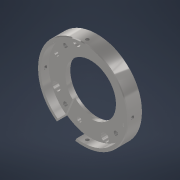
# Autodesk Inventor part: 006
Saved by Autodesk Inventor 2022 (Build 260153000, 153)
## iProperties
Created: 2021-11-05
Part Number: 006
Material: Stainless Steel, 440C
Document SubType Name: Modeling
Designer: vinicius.miguel
Density: 7.75 g/cm^3
Appearance: Semi-Polished
Mass: 959.118 g
Surface Area: 466.738 cm^2
Volume: 123.757 cm^3
Author: vinicius.miguel
Autodesk Inventor part; units mm, degrees
ref_plane "XY Plane" through (0, 0, 0) normal (0, 0, 1) x (1, 0, 0)
sketch "Sketch1" plane through (0, 0, 0) normal (0, 1, 0) x (-1, 0, 0)
  line L0 (0, 0) -> (0, -51.1103) construction
  line L1 (-37.5, -17) -> (-40, -17)
  line L2 (-40, -17) -> (-40, -22)
  line L3 (-40, -22) -> (-67, -22)
  line L4 (-67, -22) -> (-67, 0)
  line L5 (-67, 0) -> (-62, 0)
  line L6 (-62, 0) -> (-62, -12)
  line L7 (-62, -12) -> (-37.5, -12)
  line L8 (-37.5, -12) -> (-37.5, -17)
  dimension "d0" = 75
  dimension "d1" = 80
  dimension "d2" = 5
  dimension "d3" = 124
  dimension "d4" = 134
  dimension "d5" = 12
  dimension "d8" = 5
  constraints: 18 end point, 6 perpendicular, 1 horizontal, 1 horizontal alignment, 1 vertical
  measures "d0" diameter of L8 L0
  measures "d1" diameter of L2 L0
  measures "d2" distance of L1.end L2.end
  measures "d3" diameter of L6 L0
  measures "d4" diameter of L4 L0
  measures "d5" distance of L5.end L6.end
  measures "d8" distance of L7.end L1.start
revolve "Revolution1" add sketch "Sketch1" angle 360 about axis through (0, 0, 0) along (0, 0, -1)
sketch "Sketch2" plane through (0, 0, -22) normal (0, 0, -1) x (-1, 0, 0)
  line L0 (0, 0) -> (103.3512, 0)
  line L1 (0, 0) -> (37.4767, 37.4767)
  circle A0 centre (37.4767, 37.4767) radius 7.75
  circle A1 centre (0, 0) radius 44.45 projected
  dimension "d10" = 53
  dimension "d72" = 45
  dimension "d79" = 15.5
  constraints: 4 end point, 1 centre point, 1 coincident, 1 horizontal
  measures "d10" distance of L1.end L0.start
  measures "d72" angle of L0 L1
  measures "d79" diameter of A0
hole "Hole1" at (-37.4767, 37.4767, -22) direction (0, 0, 1) diameter 6.647 depth 22.2 tip angle 118 thread size "M8x1.25" class "6H" standard "ANSI Metric M Profile"
pattern_circular "Circular Pattern1" count 4 over 360 about axis through (0, 0, -11) along (0, 0, 1) of "Hole1"
sketch "Sketch3" plane through (0, 0, -22) normal (0, 0, -1) x (-1, 0, 0)
  circle A0 centre (0, 0) radius 62 projected
  line L0 (62, 0) -> (0, 0)
  line L1 (50.8134, -21.0476) -> (0, 0)
  point P0 (47.6314, 27.5)
  point P1 (0, 55)
  point P2 (-47.6314, 27.5)
  point P3 (-47.6314, -27.5)
  point P4 (0, -55)
  dimension "d25" = 55
  dimension "d37" = 22.5
  constraints: 4 end point, 1 horizontal, 1 horizontal alignment
  measures "d25" distance of point (0, 0) L1.start
  measures "d37" angle of L0 L1
hole "Hole2" at (-50.8134, -21.0476, -22) direction (0, 0, 1) diameter 7 end through all clearance for "Countersunk Flat Head Screw DIN EN ISO 2009" size "M6" standard "DIN"
pattern_circular "Circular Pattern2" count 8 over 360 about axis through (0, 0, -11) along (0, 0, 1) of "Hole2"
chamfer "Chamfer1" distance 1 angle 45 2 edges at (-67, 0, -22) (-67, 0, 0)
chamfer "Chamfer2" distance 0.2 angle 45 1 edges at (-40, 0, -22)
ref_plane "Work Plane1" through (-67, 0, -11) normal (1, 0, 0) x (0, 1, 0)
ref_plane "Work Plane2" through (0, 67, -11) normal (0, 1, 0) x (-1, 0, 0)
sketch "Sketch4" plane through (0, 67, -11) normal (0, 1, 0) x (-1, 0, 0)
  line L0 (66, -11) -> (-66, -11) projected
  point P0 (0, 11)
  point P1 (0, 4)
  point P2 (0, -11)
  dimension "d44" = 15
  constraints: 1 midpoint, 1 vertical alignment
  measures "d44" distance from line of point (0, 4) L0
hole "Hole3" at (0, 67, -7) direction (0, -1, 0) diameter 4.917 end through all thread size "M6x1" class "6H" standard "ANSI Metric M Profile"
sketch "Sketch5" plane through (-67, 0, -11) normal (1, 0, 0) x (0, 1, 0)
  line L0 (66, -11) -> (-66, -11) projected
  point P0 (0, 11)
  point P1 (0, 4)
  point P2 (0, -11)
  dimension "d52" = 15
  constraints: 1 midpoint, 1 vertical alignment
  measures "d52" distance from line of point (0, 4) L0
hole "Hole4" at (-67, 0, -7) direction (1, 0, 0) diameter 4.917 end through all thread size "M6x1" class "6H" standard "ANSI Metric M Profile"
sketch "Sketch6" plane through (0, 0, 0) normal (0, 0, 1) x (1, 0, 0)
  line L0 (-13.8582, 5.7403) -> (-52.1265, -86.6477)
  line L1 (-52.1265, -86.6477) -> (-24.4102, -98.1282)
  line L2 (-24.4102, -98.1282) -> (13.8582, -5.7403)
  line L3 (13.8582, -5.7403) -> (-13.8582, 5.7403)
  line L4 (0, 0) -> (26.9021, 0)
  dimension "d60" = 30
  dimension "d61" = 100
  dimension "d65" = 22.5
  constraints: 10 end point, 2 parallel, 1 coincident, 1 horizontal, 1 midpoint, 1 perpendicular
  measures "d60" distance of L0.end L1.end
  measures "d61" distance of L0.start L0.end
  measures "d65" angle of L3 L4
extrude "Extrusion1" cut sketch "Sketch6" against normal blind 16
sketch "Sketch8" plane through (0, 0, -22) normal (0, 0, -1) x (-1, 0, 0)
  circle A0 centre (-50.8134, 21.0476) radius 3.5 projected
  circle A1 centre (-21.0476, -50.8134) radius 3.5 projected
  circle A2 centre (50.8134, -21.0476) radius 3.5 projected
  circle A3 centre (21.0476, 50.8134) radius 3.5 projected
  circle A4 centre (-50.8134, 21.0476) radius 6
  circle A5 centre (21.0476, 50.8134) radius 6
  circle A6 centre (-21.0476, -50.8134) radius 6
  circle A7 centre (50.8134, -21.0476) radius 6
  point P0 (0, 0)
  dimension "d76" = 12
  constraints: 4 centre point, 3 equal radius
  measures "d76" diameter of A6
extrude "Extrusion3" cut sketch "Sketch8" against normal through all contours A0 | A4 | A5 | A6 | A7
body "Solid1"
